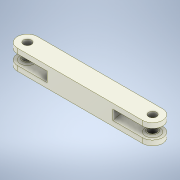
# Autodesk Inventor part: LinkB
Saved by Autodesk Inventor 2022 (Build 260153000, 153)
## iProperties
Created: 2021-11-22
Part Number: LinkB
Material: Plástico ABS
Document SubType Name: Modeling
Designer: JK
Density: 1.06 g/cm^3
Appearance: Suave - Marfil
Author: JK
Autodesk Inventor part; units mm, degrees
ref_plane "YZ Plane" through (0, 0, 0) normal (1, 0, 0) x (0, 1, 0)
ref_plane "XZ Plane" through (0, 0, 0) normal (0, 1, 0) x (-1, 0, 0)
ref_plane "XY Plane" through (0, 0, 0) normal (0, 0, 1) x (1, 0, 0)
sketch "Boceto1" plane through (0, 0, 0) normal (0, 1, 0) x (-1, 0, 0)
  line L0 (-25, 4) -> (25, 4)
  line L1 (25, 4) -> (25, -4)
  line L2 (25, -4) -> (-25, -4)
  line L3 (-25, -4) -> (-25, 4)
  line L4 (-25, 4) -> (25, -4) construction
  line L5 (25, 4) -> (-25, -4) construction
  circle A0 centre (25, 0) radius 4
  circle A1 centre (25, 0) radius 1.6
  circle A2 centre (-25, 0) radius 4
  circle A3 centre (-25, 0) radius 1.6
  point P0 (0, 0)
  point P1 (25, 4)
  point P2 (-25, 4)
  dimension "d0" = 8
  dimension "d1" = 3.2
  dimension "d2" = 3.2
  dimension "d15" = 50
  constraints: 12 end point, 4 midpoint, 2 centre point, 2 coincident, 2 horizontal, 2 parallel, 1 perpendicular, 6 other
  measures "d1" diameter of A1
  measures "d2" diameter of A3
  measures "d15" distance of L0.start L0.end
extrude "Extrusión1" add sketch "Boceto1" along normal blind 8 contours A2 L3 A3 | L0 A0 L2 A2 | L3 A3 A2 | A0 L1 A1 | L1 A1 A0
ref_plane "Plano de trabajo1" through (0, 4, 0) normal (0, -1, 0) x (1, 0, 0)
sketch "Boceto2" plane through (0, 4, 0) normal (0, -1, 0) x (1, 0, 0)
  circle A0 centre (25, 0) radius 1.6 projected
  circle A1 centre (25, 0) radius 12.5
  circle A2 centre (-25, 0) radius 1.6 projected
  circle A3 centre (-25, 0) radius 12.5
  point P0 (0, 0)
  dimension "d5" = 25
  dimension "d23" = 25
  constraints: 2 centre point, 2 coincident
  measures "d5" diameter of A1
  measures "d23" diameter of A3
extrude "Extrusión2" cut sketch "Boceto2" along normal mid plane 4
sketch "Boceto3" plane through (0, 2, 0) normal (0, 1, 0) x (1, 0, 0)
  circle A0 centre (25, 0) radius 1.6 projected
  circle A1 centre (25, 0) radius 2
  circle A2 centre (-25, 0) radius 1.6 projected
  circle A3 centre (-25, 0) radius 2
  point P0 (0, 0)
  dimension "d9" = 4
  dimension "d24" = 4
  constraints: 2 centre point, 2 coincident
  measures "d9" diameter of A1
  measures "d24" diameter of A3
extrude "Extrusión3" add sketch "Boceto3" along normal up to surface (4 mm away)
sketch "Boceto4" plane through (-25, 0, 4) normal (0, 0, 1) x (1, 0, 0)
  line L0 (38.1573, 5.5) -> (52.3985, 5.5)
  line L1 (52.3985, 5.5) -> (52.3985, 2.5)
  line L2 (52.3985, 2.5) -> (38.1573, 2.5)
  line L3 (38.1573, 2.5) -> (38.1573, 5.5)
  line L4 (38.1573, 5.5) -> (52.3985, 2.5) construction
  line L5 (52.3985, 5.5) -> (38.1573, 2.5) construction
  line L6 (38.1573, 2) -> (38.1573, 6) projected
  line L7 (11.8427, 2) -> (11.8427, 6) projected
  line L8 (-10.1369, 2.5) -> (11.8427, 2.5)
  line L9 (11.8427, 2.5) -> (11.8427, 5.5)
  line L10 (11.8427, 5.5) -> (-10.1369, 5.5)
  line L11 (-10.1369, 5.5) -> (-10.1369, 2.5)
  line L12 (-10.1369, 2.5) -> (11.8427, 5.5) construction
  line L13 (11.8427, 2.5) -> (-10.1369, 5.5) construction
  point P0 (25, 0)
  point P1 (45.2779, 4)
  point P2 (45.2779, 4)
  point P3 (38.1573, 4)
  point P4 (0.8529, 4)
  dimension "d12" = 3
  constraints: 24 end point, 6 midpoint, 4 parallel, 3 collinear, 2 horizontal, 2 perpendicular, 1 horizontal alignment, 1 point on line
  measures "d12" distance between parallel lines of L2 L0
extrude "Extrusión4" cut sketch "Boceto4" against normal through all
fillet "Empalme2" radius 1 4 edges at (23, 2, 0) (23, 6, 0) (-27, 2, 0) (-27, 6, 0)
sketch "Boceto5" plane through (0, 0, 0) normal (0, -1, 0) x (1, 0, 0)
  circle A0 centre (-25, 0) radius 1.6 projected
  circle A1 centre (-25, 0) radius 8.75
  point P0 (0, 0)
  dimension "d16" = 17.5
  constraints: 1 centre point, 1 coincident
  measures "d16" diameter of A1
sketch "Boceto6" plane through (0, 7.5, 0) normal (0, -1, 0) x (1, 0, 0)
  circle A0 centre (-20, 0) radius 1.5 projected
  circle A1 centre (-20, 0) radius 2
  circle A2 centre (-20, 0) radius 1.5 projected
  point P0 (0, 0)
  dimension "d19" = 4
  constraints: 1 centre point, 1 coincident
  measures "d19" diameter of A1
